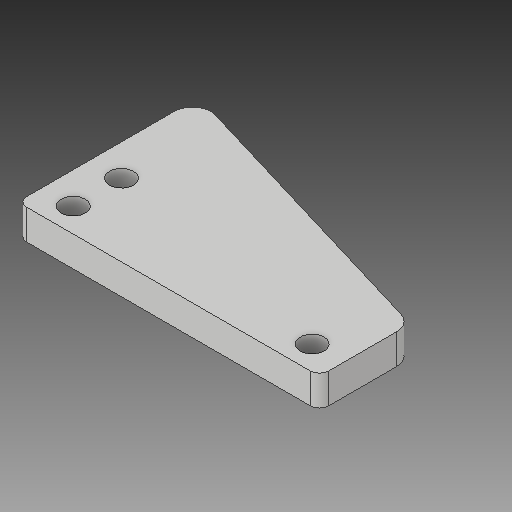
# Autodesk Inventor part: TrackSypport
Saved by Autodesk Inventor 2017 (Build 210142000, 142)
## iProperties
Created: 2016-12-06
Part Number: TrackSypport
Material: Generic
Document SubType Name: Modeling
Designer: umr
Density: 1 g/cm^3
Appearance: Default
Author: umr
Autodesk Inventor part; units mm, degrees
ref_plane "YZ Plane" through (0, 0, 0) normal (1, 0, 0) x (0, 1, 0)
ref_plane "XZ Plane" through (0, 0, 0) normal (0, 1, 0) x (-1, 0, 0)
ref_plane "XY Plane" through (0, 0, 0) normal (0, 0, 1) x (1, 0, 0)
sketch "Sketch1" plane through (0, 0, 0) normal (0, 1, 0) x (-1, 0, 0)
  line L0 (3, 0) -> (97, 0)
  line L1 (100, -3) -> (100, -51.9358)
  line L2 (92.2759, -57.6828) -> (4.2759, -31.2828)
  line L3 (0, -25.5358) -> (0, -3)
  arc A0 (92.2759, -57.6828) -> (100, -51.9358) centre (94, -51.9358) ccw
  arc A1 (0, -25.5358) -> (4.2759, -31.2828) centre (6, -25.5358) ccw
  arc A2 (100, -3) -> (97, 0) centre (97, -3) ccw
  arc A3 (3, 0) -> (0, -3) centre (3, -3) ccw
  point P0 (0, 0)
  point P1 (100, 0)
  point P2 (100, -60)
  point P3 (0, -30)
  dimension "d0" = 100
  dimension "d1" = 60
  dimension "d2" = 30
  dimension "d3" = 6
  dimension "d4" = 6
  dimension "d5" = 3
  constraints: 8 end point, 8 point on circle, 8 point on line, 8 tangent, 4 centre point, 1 equal radius, 1 horizontal, 1 parallel, 1 vertical
  measures "d0" distance of point (0, 0) point (100, 0)
  measures "d1" distance of point (100, 0) point (100, -60)
  measures "d2" distance of point (0, -30) point (0, 0)
  measures "d3" radius of A0
  measures "d4" radius of A1
  measures "d5" radius of A2
extrude "Extrusion1" add sketch "Sketch1" along normal blind 10
sketch "Sketch2" plane through (0, 0, 0) normal (0, -1, 0) x (1, 0, 0)
  circle A0 centre (-10.4444, -8) radius 4
  circle A1 centre (-89.5556, -8) radius 4
  line L0 (-100, -51.9358) -> (-100, -3) projected
  arc A2 (-100, -51.9358) -> (-92.2759, -57.6828) centre (-94, -51.9358) ccw projected
  line L1 (-4.2759, -31.2828) -> (-92.2759, -57.6828) projected
  arc A3 (-4.2759, -31.2828) -> (0, -25.5358) centre (-6, -25.5358) ccw projected
  line L2 (0, -3) -> (0, -25.5358) projected
  arc A4 (0, -3) -> (-3, 0) centre (-3, -3) ccw projected
  line L3 (-97, 0) -> (-3, 0) projected
  arc A5 (-97, 0) -> (-100, -3) centre (-97, -3) ccw projected
  circle A6 centre (-89.5556, -24) radius 4
  point P0 (0, 0)
  dimension "d8" = 8
  dimension "d9" = 8
  dimension "d10" = 94
  dimension "d11" = 10.4444
  dimension "d12" = 10.4444
  dimension "d13" = 22.5358
  dimension "d14" = 8
  dimension "d15" = 8
  dimension "d18" = 8
  dimension "d19" = 16
  dimension "d20" = 10.4444
  constraints: 3 centre point
  measures "d8" diameter of A0
  measures "d9" diameter of A1
  measures "d10" distance of L3.start L3.end
  measures "d11" distance from line of L2 A0.centre
  measures "d12" distance from line of A1.centre L0
  measures "d13" distance of L2.start L2.end
  measures "d14" distance from line of L3 A0.centre
  measures "d15" distance from line of L3 A1.centre
  measures "d18" diameter of A6
  measures "d19" distance of A1.centre A6.centre
  measures "d20" distance from line of L0 A6.centre
extrude "Extrusion2" cut sketch "Sketch2" against normal through all contours A0 | A1 | A6
equation "\"d1\" = 0.6 * d0"
equation "\"d2\" = 0.5 * d1"
equation "\"d3\" = 0.2 * d2"
equation "\"d4\" = d3"
equation "\"d5\" = 0.5 * d3"
equation "\"d9\" = d8"
equation "\"d11\" = 0.111111 * d10"
equation "\"d12\" = d11"
equation "\"d14\" = d8"
equation "\"d15\" = d8"
equation "\"d18\" = d9"
equation "\"d19\" = 2 * d9"
equation "\"d20\" = d12"
body "Solid1"
